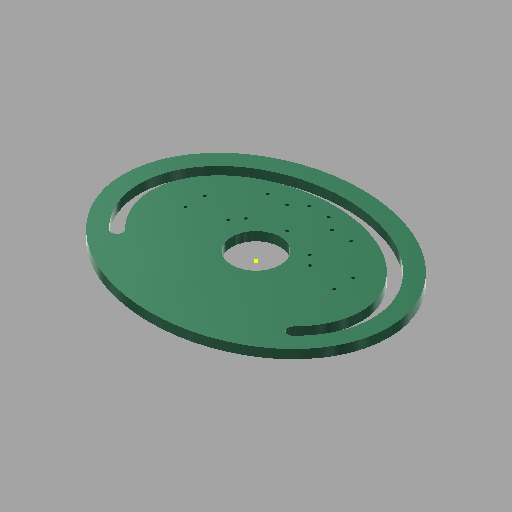
# Autodesk Inventor part: 24_0497_002
Saved by Autodesk Inventor 2024.3 (Build 283343000, 343)
## iProperties
Created: 2024-05-28
Part Number: 24_0497_002
Material: LCP-Kunststoff
Document SubType Name: Modeling
Designer: Vogel
Density: 1.626 g/cm^3
Appearance: Glatt - Dunkelseegrün
Author: Vogel
Autodesk Inventor part; units mm, degrees
ref_plane "YZ Plane" through (0, 0, 0) normal (1, 0, 0) x (0, 1, 0)
ref_plane "XZ Plane" through (0, 0, 0) normal (0, 1, 0) x (-1, 0, 0)
ref_plane "XY Plane" through (0, 0, 0) normal (0, 0, 1) x (1, 0, 0)
sketch "Skizze1" plane through (0, 0, 0) normal (0, 0, 1) x (1, 0, 0)
  line L0 (-210, 0) -> (210, 0) projected
  line L1 (0, -168) -> (0, 168) projected
  ellipse E0 centre (0, 0) end of major axis (-150, 0) minor radius 120
  line L2 (0, 120) -> (0, -120) construction
  line L3 (-150, 0) -> (150, 0) construction
  dimension "d0" = 300
  dimension "d1" = 240
  constraints: 4 end point, 4 point on line, 1 coincident, 6 other
  measures "d0" distance of L3.start L3.end
  measures "d1" distance of L2.start L2.end
extrude "Extrusion1" add sketch "Skizze1" along normal blind 10
sketch "Skizze2" plane through (0, 0, 10) normal (0, 0, 1) x (1, 0, 0)
  ellipse E0 centre (0, 0) end of major axis (-150, 0) minor radius 120 projected
  line L0 (0, -168) -> (0, 168) projected
  line L1 (-210, 0) -> (210, 0) projected
  line L2 (-131.5, 0) -> (131.5, 0)
  line L3 (0, 101.5) -> (0, -101.5)
  ellipse E1 centre (0, 0) end of major axis (-131.5, 0) minor radius 101.5
  line L4 (0, 0) -> (-105.3012, -60.7957) construction
  line L5 (0, 0) -> (105.3012, -60.7957) construction
  ellipse E2 centre (0, 0) end of major axis (118.5, 0) minor radius 88.5
  line L6 (0, 0) -> (80.349, 80.349) construction
  line L7 (80.349, 80.349) -> (73.764, 69.2632)
  line L8 (67.3414, 73.0783) -> (84.3123, 62.9974)
  arc A0 (94.9826, -52.9176) -> (105.1165, -60.6891) centre (99.5391, -57.469) ccw
  arc A1 (-105.1165, -60.6891) -> (-94.9826, -52.9176) centre (-99.5391, -57.469) ccw
  point P0 (0, 120)
  point P1 (150, 0)
  point P2 (-150, 0)
  point P3 (0, -120)
  point P4 (118.5, 0)
  point P5 (-96, 0)
  point P6 (0, 88.5)
  point P7 (-104.0928, -62.0231)
  point P8 (104.0928, -62.0231)
  dimension "d7" = 18.5
  dimension "d8" = 18.5
  dimension "d9" = 31.5
  dimension "d10" = 31.5
  dimension "d11" = 45
  dimension "d12" = 90
  dimension "d13" = 12.8941
  dimension "d14" = 30
  dimension "d15" = 30
  constraints: 16 point on line, 14 end point, 7 coincident, 4 point on circle, 2 centre point, 2 horizontal, 2 symmetric about line, 24 other
  measures "d7" distance of point (0, 120) L3.start
  measures "d8" distance of L2.end point (150, 0)
  measures "d9" distance of point (0, 120) point (0, 88.5)
  measures "d10" distance of point (150, 0) point (118.5, 0)
  measures "d11" angle of L6 L1
  measures "d12" angle of L8 L7
  measures "d13" distance of L6.end L7.end
  measures "d14" angle of L2 L5
  measures "d15" angle of L2 L4
extrude "Extrusion2" cut sketch "Skizze2" against normal through all contours E1 L0 E2 L1 | L1 E2 A1 E1 | E1 L7 E2 L0 | E1 A0 E2 L1 | L1 E2 L7 E1
sketch "Skizze4" plane through (0, 0, 10) normal (0, 0, 1) x (1, 0, 0)
  circle A0 centre (0, 0) radius 27.5 projected
extrude "Extrusion4" cut sketch "Skizze4" against normal through all
sketch "Skizze5" plane through (0, 0, 10) normal (0, 0, 1) x (1, 0, 0)
  circle A0 centre (44.6817, 16.1402) radius 2.2 projected
  circle A1 centre (81.576, 6.678) radius 2.2 projected
  circle A2 centre (81.1696, 28.4843) radius 2.2 projected
  circle A3 centre (34.1537, 26.537) radius 2.2 projected
  circle A4 centre (-1.9423, 37.1246) radius 2.2 projected
  circle A5 centre (-37.5824, 25.8884) radius 2.2 projected
  circle A6 centre (-46.0331, 14.7062) radius 2.2 projected
  circle A7 centre (-82.7479, 3.0545) radius 2.1998 projected
  circle A8 centre (-82.7419, 24.8643) radius 2.1999 projected
  circle A9 centre (-49.2342, 62.6033) radius 2.2 projected
  circle A10 centre (-27.4241, 62.5973) radius 2.2 projected
  circle A11 centre (-13.5942, 73.8395) radius 2.2001 projected
  circle A12 centre (8.2159, 73.8333) radius 2.2 projected
  circle A13 centre (22.5018, 63.2519) radius 2.2 projected
  circle A14 centre (44.3119, 63.2458) radius 2.2 projected
  point P0 (0, 0)
  constraints: 15 coincident
hole "Bohrung1" at (81.576, 6.678, 10) at (81.1696, 28.4843, 10) at (44.6817, 16.1402, 10) at (34.1537, 26.537, 10) at (-1.9423, 37.1246, 10) at (8.2159, 73.8333, 10) at (-13.5942, 73.8395, 10) at (22.5018, 63.2519, 10) at (44.3119, 63.2458, 10) at (-27.4241, 62.5973, 10) at (-49.2342, 62.6033, 10) at (-37.5824, 25.8884, 10) at (-46.0331, 14.7062, 10) at (-82.7479, 3.0545, 10) at (-82.7419, 24.8643, 10) direction (0, 0, -1) diameter 3.242 end through all thread size "M4x0.7" class "6H" standard "ISO Metric profile"
sketch "Skizze6" plane through (0, 0, 0) normal (0, 0, -1) x (-1, 0, 0)
  point P0 (0, 0)
equation "\"d8\" = d7"
equation "\"d10\" = d9"
